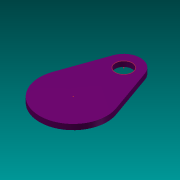
# Autodesk Inventor part: Key Fob
Saved by Autodesk Inventor 2015 (Build 190159000, 159)
## iProperties
Created: 2015-06-23
Part Number: Key Fob
Material: ABS Plastic
Document SubType Name: Modeling
Designer: Sawaiz Syed
Density: 1.06 g/cm^3
Appearance: Smooth - Purple
Author: Sawaiz Syed
Autodesk Inventor part; units mm, degrees
ref_plane "YZ Plane" through (0, 0, 0) normal (1, 0, 0) x (0, 1, 0)
ref_plane "XZ Plane" through (0, 0, 0) normal (0, 1, 0) x (-1, 0, 0)
ref_plane "XY Plane" through (0, 0, 0) normal (0, 0, 1) x (1, 0, 0)
sketch "Sketch1" plane through (0, 0, 0) normal (0, 0, 1) x (1, 0, 0)
  circle A0 centre (0, 0) radius 10
  circle A1 centre (0, 15) radius 5
  line L0 (0, 0) -> (0, 15)
  line L1 (-4.714, 16.6667) -> (-9.4281, 3.3333)
  line L2 (4.714, 16.6667) -> (9.4281, 3.3333)
  dimension "d0" = 20
  dimension "d1" = 10
  constraints: 6 end point, 5 tangent, 4 point on circle, 2 centre point, 1 coincident, 1 vertical
  measures "d0" diameter of A0
  measures "d1" diameter of A1
extrude "Extrusion1" add sketch "Sketch1" along normal blind 1.6
sketch "Sketch2" plane through (0, 0, 1.6) normal (0, 0, 1) x (1, 0, 0)
  arc A0 (-9.4281, 3.3333) -> (9.4281, 3.3333) centre (0, 0) ccw projected
  line L0 (9.4281, 3.3333) -> (4.714, 16.6667) projected
  arc A1 (4.714, 16.6667) -> (-4.714, 16.6667) centre (0, 15) ccw projected
  line L1 (-4.714, 16.6667) -> (-9.4281, 3.3333) projected
  constraints: 1 coincident
hole "Hole1" at (0, 15, 1.6) direction (0, 0, -1) diameter 5 end through all
sketch "Sketch3" plane through (0, 0, 1.6) normal (0, 0, 1) x (1, 0, 0)
  circle A0 centre (0, 15) radius 2.5 projected
  point P0 (0, 0)
body "Solid1"
